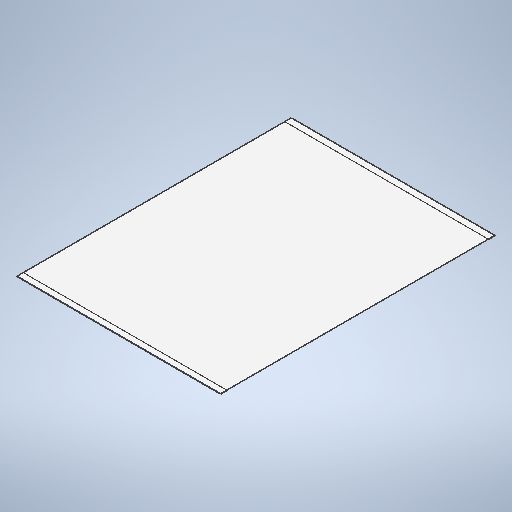
# Autodesk Inventor part: field_plate_SUS4301
Saved by Autodesk Inventor 2025 (Build 290162000, 162)
## iProperties
Created: 2026-02-16
Part Number: field_plate_SUS4301
Material: 一般
Document SubType Name: Modeling
Designer: sooo1
Density: 1 g/cm^3
Appearance: 既定(1)
Author: sooo1
Autodesk Inventor part; units mm, degrees
ref_plane "YZ Plane" through (0, 0, 0) normal (1, 0, 0) x (0, 1, 0)
ref_plane "XZ Plane" through (0, 0, 0) normal (0, 1, 0) x (-1, 0, 0)
ref_plane "XY Plane" through (0, 0, 0) normal (0, 0, 1) x (1, 0, 0)
sketch "スケッチ1" plane through (0, 0, 0) normal (0, 1, 0) x (-1, 0, 0)
  line L0 (148.5, 200.09) -> (-148.5, 200.09)
  line L1 (-148.5, 200.09) -> (-148.5, -200.09)
  line L2 (-148.5, -200.09) -> (148.5, -200.09)
  line L3 (148.5, -200.09) -> (148.5, 200.09)
  line L4 (148.5, 200.09) -> (-148.5, -200.09) construction
  line L5 (-148.5, 200.09) -> (148.5, -200.09) construction
  line L6 (-148.5, 190.77) -> (148.5, 190.77)
  line L7 (-207.9, 0) -> (207.9, 0) construction
  line L8 (-148.5, -190.77) -> (148.5, -190.77)
  line L9 (-148.5, 200) -> (148.5, 200)
  line L10 (-148.5, -200) -> (148.5, -200)
  point P0 (0, 0)
  point P1 (-148.5, -200)
  point P2 (-148.5, -190.77)
  dimension "d1" = 297
  dimension "d4" = 9.32
  dimension "d5" = 0.09
  dimension "d10" = 400
  constraints: 20 end point, 4 point on line, 4 symmetric about line, 3 perpendicular, 2 midpoint, 2 parallel, 1 horizontal
  measures "d1" distance of L0.start L0.end
  measures "d4" distance between parallel lines of L0 L6
  measures "d5" distance between parallel lines of L0 L9
  measures "d10" distance between parallel lines of L10 L9
extrude "押し出し1" add sketch "スケッチ1" along normal blind 0.09
extrude "押し出し2" add sketch "スケッチ1" against normal blind 0.5 contours L3 L9 L1 L0 | L3 L2 L1 L10
extrude "押し出し3" add sketch "スケッチ1" against normal blind 0.09 from surface at -0.5 contours L3 L9 L1 L0 | L3 L6 L1 L9 | L3 L10 L1 L8 | L3 L2 L1 L10
